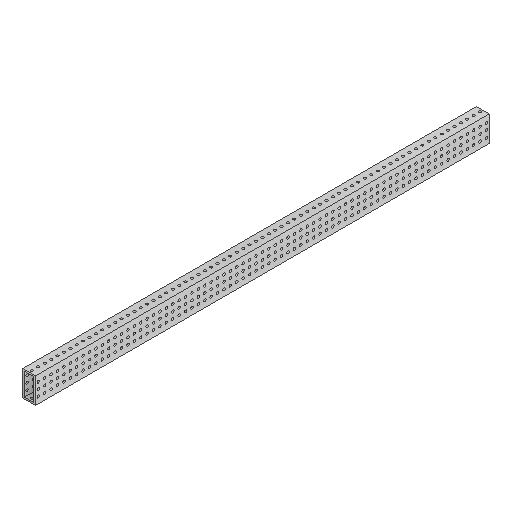
# Autodesk Inventor part: Forja - Base Chassi
Saved by Autodesk Inventor 2027.1 (Build 311270010, 270A)
## iProperties
Created: 2026-05-13
Part Number: Forja - Base Chassi
Material: Genérico
Document SubType Name: Modeling
Designer: djair.oliveira
Density: 1 g/cm^3
Appearance: Padrão
Author: djair.oliveira
Autodesk Inventor part; units mm, degrees
ref_plane "YZ Plane" through (0, 0, 0) normal (1, 0, 0) x (0, 1, 0)
ref_plane "XZ Plane" through (0, 0, 0) normal (0, 1, 0) x (-1, 0, 0)
ref_plane "XY Plane" through (0, 0, 0) normal (0, 0, 1) x (1, 0, 0)
sketch "Esboço1" plane through (0, 0, 0) normal (0, 0, 1) x (1, 0, 0)
  line L0 (12.7, -25.4) -> (-12.7, -25.4)
  line L1 (-12.7, -25.4) -> (-12.7, 25.4)
  line L2 (-12.7, 25.4) -> (12.7, 25.4)
  line L3 (12.7, 25.4) -> (12.7, -25.4)
  line L4 (12.7, -25.4) -> (-12.7, 25.4) construction
  line L5 (-12.7, -25.4) -> (12.7, 25.4) construction
  line L6 (9.525, -22.225) -> (-9.525, -22.225)
  line L7 (-9.525, -22.225) -> (-9.525, 22.225)
  line L8 (-9.525, 22.225) -> (9.525, 22.225)
  line L9 (9.525, 22.225) -> (9.525, -22.225)
  line L10 (9.525, -22.225) -> (-9.525, 22.225) construction
  line L11 (-9.525, -22.225) -> (9.525, 22.225) construction
  point P0 (0, 0)
  dimension "d1" = 3.175
  dimension "d2" = 3.175
  dimension "d3" = 25.4
  dimension "d4" = 50.8
  constraints: 24 end point, 4 midpoint, 4 parallel, 2 horizontal, 2 perpendicular
  measures "d1" distance between parallel lines of L1 L7
  measures "d2" distance between parallel lines of L2 L8
  measures "d3" distance of L1.end L2.end
  measures "d4" distance of L2.end L0.start
extrude "Extrusão1" add sketch "Esboço1" along normal blind 900
sketch "Esboço2" plane through (-12.7, 25.4, 0) normal (0, 1, 0) x (1, 0, 0)
  circle A0 centre (12.7, -450) radius 2.5
  line L0 (0, 0) -> (0, -900) projected
  line L1 (25.4, -900) -> (0, -900) projected
  line L2 (25.4, 0) -> (0, 0) projected
  circle A1 centre (12.7, -462.7) radius 2.5
  circle A2 centre (12.7, -437.3) radius 2.5
  circle A3 centre (12.7, -475.4) radius 2.5
  circle A4 centre (12.7, -424.6) radius 2.5
  circle A5 centre (12.7, -488.1) radius 2.5
  circle A6 centre (12.7, -411.9) radius 2.5
  circle A7 centre (12.7, -500.8) radius 2.5
  circle A8 centre (12.7, -399.2) radius 2.5
  circle A9 centre (12.7, -513.5) radius 2.5
  circle A10 centre (12.7, -386.5) radius 2.5
  circle A11 centre (12.7, -526.2) radius 2.5
  circle A12 centre (12.7, -373.8) radius 2.5
  circle A13 centre (12.7, -538.9) radius 2.5
  circle A14 centre (12.7, -361.1) radius 2.5
  circle A15 centre (12.7, -551.6) radius 2.5
  circle A16 centre (12.7, -348.4) radius 2.5
  circle A17 centre (12.7, -564.3) radius 2.5
  circle A18 centre (12.7, -335.7) radius 2.5
  circle A19 centre (12.7, -577) radius 2.5
  circle A20 centre (12.7, -323) radius 2.5
  circle A21 centre (12.7, -589.7) radius 2.5
  circle A22 centre (12.7, -310.3) radius 2.5
  circle A23 centre (12.7, -602.4) radius 2.5
  circle A24 centre (12.7, -297.6) radius 2.5
  circle A25 centre (12.7, -615.1) radius 2.5
  circle A26 centre (12.7, -284.9) radius 2.5
  circle A27 centre (12.7, -627.8) radius 2.5
  circle A28 centre (12.7, -272.2) radius 2.5
  circle A29 centre (12.7, -640.5) radius 2.5
  circle A30 centre (12.7, -259.5) radius 2.5
  circle A31 centre (12.7, -653.2) radius 2.5
  circle A32 centre (12.7, -246.8) radius 2.5
  circle A33 centre (12.7, -665.9) radius 2.5
  circle A34 centre (12.7, -234.1) radius 2.5
  circle A35 centre (12.7, -678.6) radius 2.5
  circle A36 centre (12.7, -221.4) radius 2.5
  circle A37 centre (12.7, -691.3) radius 2.5
  circle A38 centre (12.7, -208.7) radius 2.5
  circle A39 centre (12.7, -704) radius 2.5
  circle A40 centre (12.7, -196) radius 2.5
  circle A41 centre (12.7, -716.7) radius 2.5
  circle A42 centre (12.7, -183.3) radius 2.5
  circle A43 centre (12.7, -729.4) radius 2.5
  circle A44 centre (12.7, -170.6) radius 2.5
  circle A45 centre (12.7, -742.1) radius 2.5
  circle A46 centre (12.7, -157.9) radius 2.5
  circle A47 centre (12.7, -754.8) radius 2.5
  circle A48 centre (12.7, -145.2) radius 2.5
  circle A49 centre (12.7, -767.5) radius 2.5
  circle A50 centre (12.7, -132.5) radius 2.5
  circle A51 centre (12.7, -780.2) radius 2.5
  circle A52 centre (12.7, -119.8) radius 2.5
  circle A53 centre (12.7, -792.9) radius 2.5
  circle A54 centre (12.7, -107.1) radius 2.5
  circle A55 centre (12.7, -805.6) radius 2.5
  circle A56 centre (12.7, -94.4) radius 2.5
  circle A57 centre (12.7, -818.3) radius 2.5
  circle A58 centre (12.7, -81.7) radius 2.5
  circle A59 centre (12.7, -831) radius 2.5
  circle A60 centre (12.7, -69) radius 2.5
  circle A61 centre (12.7, -843.7) radius 2.5
  circle A62 centre (12.7, -56.3) radius 2.5
  circle A63 centre (12.7, -856.4) radius 2.5
  circle A64 centre (12.7, -43.6) radius 2.5
  circle A65 centre (12.7, -869.1) radius 2.5
  circle A66 centre (12.7, -30.9) radius 2.5
  circle A67 centre (12.7, -881.8) radius 2.5
  circle A68 centre (12.7, -18.2) radius 2.5
  circle A69 centre (12.7, -894.5) radius 2.5
  circle A70 centre (12.7, -5.5) radius 2.5
  point P0 (12.7, 0)
  point P1 (12.7, -900)
  point P2 (12.7, 0)
  point P3 (12.7, 0)
  dimension "d7" = 5
  dimension "d8" = 12.7
  dimension "d9" = 900
  dimension "d10" = 450
  dimension "d13" = 12.7
  constraints: 71 centre point, 3 midpoint, 1 vertical, 140 other
  measures "d7" diameter of A0
  measures "d8" distance from line of L0 A0.centre
  measures "d9" distance of point (12.7, -900) point (12.7, 0)
  measures "d10" distance of point (12.7, 0) A0.centre
  measures "d13" distance of A0.centre A1.centre
extrude "Extrusão2" cut sketch "Esboço2" against normal up to surface (50.8 mm away)
sketch "Esboço3" plane through (12.7, -25.4, 0) normal (1, 0, 0) x (0, 0, -1)
  circle A0 centre (-450, 38.1) radius 2.5
  circle A1 centre (-450, 25.4) radius 2.5
  circle A2 centre (-450, 12.7) radius 2.5
  line L0 (0, 50.8) -> (-900, 50.8) projected
  line L1 (-450, 50.8) -> (-450, 0)
  line L2 (0, 0) -> (-900, 0) projected
  circle A3 centre (-462.7, 38.1) radius 2.5
  circle A4 centre (-462.7, 25.4) radius 2.5
  circle A5 centre (-462.7, 12.7) radius 2.5
  circle A6 centre (-437.3, 38.1) radius 2.5
  circle A7 centre (-437.3, 25.4) radius 2.5
  circle A8 centre (-437.3, 12.7) radius 2.5
  circle A9 centre (-475.4, 38.1) radius 2.5
  circle A10 centre (-475.4, 25.4) radius 2.5
  circle A11 centre (-475.4, 12.7) radius 2.5
  circle A12 centre (-424.6, 38.1) radius 2.5
  circle A13 centre (-424.6, 25.4) radius 2.5
  circle A14 centre (-424.6, 12.7) radius 2.5
  circle A15 centre (-488.1, 38.1) radius 2.5
  circle A16 centre (-488.1, 25.4) radius 2.5
  circle A17 centre (-488.1, 12.7) radius 2.5
  circle A18 centre (-411.9, 38.1) radius 2.5
  circle A19 centre (-411.9, 25.4) radius 2.5
  circle A20 centre (-411.9, 12.7) radius 2.5
  circle A21 centre (-500.8, 38.1) radius 2.5
  circle A22 centre (-500.8, 25.4) radius 2.5
  circle A23 centre (-500.8, 12.7) radius 2.5
  circle A24 centre (-399.2, 38.1) radius 2.5
  circle A25 centre (-399.2, 25.4) radius 2.5
  circle A26 centre (-399.2, 12.7) radius 2.5
  circle A27 centre (-513.5, 38.1) radius 2.5
  circle A28 centre (-513.5, 25.4) radius 2.5
  circle A29 centre (-513.5, 12.7) radius 2.5
  circle A30 centre (-386.5, 38.1) radius 2.5
  circle A31 centre (-386.5, 25.4) radius 2.5
  circle A32 centre (-386.5, 12.7) radius 2.5
  circle A33 centre (-526.2, 38.1) radius 2.5
  circle A34 centre (-526.2, 25.4) radius 2.5
  circle A35 centre (-526.2, 12.7) radius 2.5
  circle A36 centre (-373.8, 38.1) radius 2.5
  circle A37 centre (-373.8, 25.4) radius 2.5
  circle A38 centre (-373.8, 12.7) radius 2.5
  circle A39 centre (-538.9, 38.1) radius 2.5
  circle A40 centre (-538.9, 25.4) radius 2.5
  circle A41 centre (-538.9, 12.7) radius 2.5
  circle A42 centre (-361.1, 38.1) radius 2.5
  circle A43 centre (-361.1, 25.4) radius 2.5
  circle A44 centre (-361.1, 12.7) radius 2.5
  circle A45 centre (-551.6, 38.1) radius 2.5
  circle A46 centre (-551.6, 25.4) radius 2.5
  circle A47 centre (-551.6, 12.7) radius 2.5
  circle A48 centre (-348.4, 38.1) radius 2.5
  circle A49 centre (-348.4, 25.4) radius 2.5
  circle A50 centre (-348.4, 12.7) radius 2.5
  circle A51 centre (-564.3, 38.1) radius 2.5
  circle A52 centre (-564.3, 25.4) radius 2.5
  circle A53 centre (-564.3, 12.7) radius 2.5
  circle A54 centre (-335.7, 38.1) radius 2.5
  circle A55 centre (-335.7, 25.4) radius 2.5
  circle A56 centre (-335.7, 12.7) radius 2.5
  circle A57 centre (-577, 38.1) radius 2.5
  circle A58 centre (-577, 25.4) radius 2.5
  circle A59 centre (-577, 12.7) radius 2.5
  circle A60 centre (-323, 38.1) radius 2.5
  circle A61 centre (-323, 25.4) radius 2.5
  circle A62 centre (-323, 12.7) radius 2.5
  circle A63 centre (-589.7, 38.1) radius 2.5
  circle A64 centre (-589.7, 25.4) radius 2.5
  circle A65 centre (-589.7, 12.7) radius 2.5
  circle A66 centre (-310.3, 38.1) radius 2.5
  circle A67 centre (-310.3, 25.4) radius 2.5
  circle A68 centre (-310.3, 12.7) radius 2.5
  circle A69 centre (-602.4, 38.1) radius 2.5
  circle A70 centre (-602.4, 25.4) radius 2.5
  circle A71 centre (-602.4, 12.7) radius 2.5
  circle A72 centre (-297.6, 38.1) radius 2.5
  circle A73 centre (-297.6, 25.4) radius 2.5
  circle A74 centre (-297.6, 12.7) radius 2.5
  circle A75 centre (-615.1, 38.1) radius 2.5
  circle A76 centre (-615.1, 25.4) radius 2.5
  circle A77 centre (-615.1, 12.7) radius 2.5
  circle A78 centre (-284.9, 38.1) radius 2.5
  circle A79 centre (-284.9, 25.4) radius 2.5
  circle A80 centre (-284.9, 12.7) radius 2.5
  circle A81 centre (-627.8, 38.1) radius 2.5
  circle A82 centre (-627.8, 25.4) radius 2.5
  circle A83 centre (-627.8, 12.7) radius 2.5
  circle A84 centre (-272.2, 38.1) radius 2.5
  circle A85 centre (-272.2, 25.4) radius 2.5
  circle A86 centre (-272.2, 12.7) radius 2.5
  circle A87 centre (-640.5, 38.1) radius 2.5
  circle A88 centre (-640.5, 25.4) radius 2.5
  circle A89 centre (-640.5, 12.7) radius 2.5
  circle A90 centre (-259.5, 38.1) radius 2.5
  circle A91 centre (-259.5, 25.4) radius 2.5
  circle A92 centre (-259.5, 12.7) radius 2.5
  circle A93 centre (-653.2, 38.1) radius 2.5
  circle A94 centre (-653.2, 25.4) radius 2.5
  circle A95 centre (-653.2, 12.7) radius 2.5
  circle A96 centre (-246.8, 38.1) radius 2.5
  circle A97 centre (-246.8, 25.4) radius 2.5
  circle A98 centre (-246.8, 12.7) radius 2.5
  circle A99 centre (-665.9, 38.1) radius 2.5
  circle A100 centre (-665.9, 25.4) radius 2.5
  circle A101 centre (-665.9, 12.7) radius 2.5
  circle A102 centre (-234.1, 38.1) radius 2.5
  circle A103 centre (-234.1, 25.4) radius 2.5
  circle A104 centre (-234.1, 12.7) radius 2.5
  circle A105 centre (-678.6, 38.1) radius 2.5
  circle A106 centre (-678.6, 25.4) radius 2.5
  circle A107 centre (-678.6, 12.7) radius 2.5
  circle A108 centre (-221.4, 38.1) radius 2.5
  circle A109 centre (-221.4, 25.4) radius 2.5
  circle A110 centre (-221.4, 12.7) radius 2.5
  circle A111 centre (-691.3, 38.1) radius 2.5
  circle A112 centre (-691.3, 25.4) radius 2.5
  circle A113 centre (-691.3, 12.7) radius 2.5
  circle A114 centre (-208.7, 38.1) radius 2.5
  circle A115 centre (-208.7, 25.4) radius 2.5
  circle A116 centre (-208.7, 12.7) radius 2.5
  circle A117 centre (-704, 38.1) radius 2.5
  circle A118 centre (-704, 25.4) radius 2.5
  circle A119 centre (-704, 12.7) radius 2.5
  circle A120 centre (-196, 38.1) radius 2.5
  circle A121 centre (-196, 25.4) radius 2.5
  circle A122 centre (-196, 12.7) radius 2.5
  circle A123 centre (-716.7, 38.1) radius 2.5
  circle A124 centre (-716.7, 25.4) radius 2.5
  circle A125 centre (-716.7, 12.7) radius 2.5
  circle A126 centre (-183.3, 38.1) radius 2.5
  circle A127 centre (-183.3, 25.4) radius 2.5
  circle A128 centre (-183.3, 12.7) radius 2.5
  circle A129 centre (-729.4, 38.1) radius 2.5
  circle A130 centre (-729.4, 25.4) radius 2.5
  circle A131 centre (-729.4, 12.7) radius 2.5
  circle A132 centre (-170.6, 38.1) radius 2.5
  circle A133 centre (-170.6, 25.4) radius 2.5
  circle A134 centre (-170.6, 12.7) radius 2.5
  circle A135 centre (-742.1, 38.1) radius 2.5
  circle A136 centre (-742.1, 25.4) radius 2.5
  circle A137 centre (-742.1, 12.7) radius 2.5
  circle A138 centre (-157.9, 38.1) radius 2.5
  circle A139 centre (-157.9, 25.4) radius 2.5
  circle A140 centre (-157.9, 12.7) radius 2.5
  circle A141 centre (-754.8, 38.1) radius 2.5
  circle A142 centre (-754.8, 25.4) radius 2.5
  circle A143 centre (-754.8, 12.7) radius 2.5
  circle A144 centre (-145.2, 38.1) radius 2.5
  circle A145 centre (-145.2, 25.4) radius 2.5
  circle A146 centre (-145.2, 12.7) radius 2.5
  circle A147 centre (-767.5, 38.1) radius 2.5
  circle A148 centre (-767.5, 25.4) radius 2.5
  circle A149 centre (-767.5, 12.7) radius 2.5
  circle A150 centre (-132.5, 38.1) radius 2.5
  circle A151 centre (-132.5, 25.4) radius 2.5
  circle A152 centre (-132.5, 12.7) radius 2.5
  circle A153 centre (-780.2, 38.1) radius 2.5
  circle A154 centre (-780.2, 25.4) radius 2.5
  circle A155 centre (-780.2, 12.7) radius 2.5
  circle A156 centre (-119.8, 38.1) radius 2.5
  circle A157 centre (-119.8, 25.4) radius 2.5
  circle A158 centre (-119.8, 12.7) radius 2.5
  circle A159 centre (-792.9, 38.1) radius 2.5
  circle A160 centre (-792.9, 25.4) radius 2.5
  circle A161 centre (-792.9, 12.7) radius 2.5
  circle A162 centre (-107.1, 38.1) radius 2.5
  circle A163 centre (-107.1, 25.4) radius 2.5
  circle A164 centre (-107.1, 12.7) radius 2.5
  circle A165 centre (-805.6, 38.1) radius 2.5
  circle A166 centre (-805.6, 25.4) radius 2.5
  circle A167 centre (-805.6, 12.7) radius 2.5
  circle A168 centre (-94.4, 38.1) radius 2.5
  circle A169 centre (-94.4, 25.4) radius 2.5
  circle A170 centre (-94.4, 12.7) radius 2.5
  circle A171 centre (-818.3, 38.1) radius 2.5
  circle A172 centre (-818.3, 25.4) radius 2.5
  circle A173 centre (-818.3, 12.7) radius 2.5
  circle A174 centre (-81.7, 38.1) radius 2.5
  circle A175 centre (-81.7, 25.4) radius 2.5
  circle A176 centre (-81.7, 12.7) radius 2.5
  circle A177 centre (-831, 38.1) radius 2.5
  circle A178 centre (-831, 25.4) radius 2.5
  circle A179 centre (-831, 12.7) radius 2.5
  circle A180 centre (-69, 38.1) radius 2.5
  circle A181 centre (-69, 25.4) radius 2.5
  circle A182 centre (-69, 12.7) radius 2.5
  circle A183 centre (-843.7, 38.1) radius 2.5
  circle A184 centre (-843.7, 25.4) radius 2.5
  circle A185 centre (-843.7, 12.7) radius 2.5
  circle A186 centre (-56.3, 38.1) radius 2.5
  circle A187 centre (-56.3, 25.4) radius 2.5
  circle A188 centre (-56.3, 12.7) radius 2.5
  circle A189 centre (-856.4, 38.1) radius 2.5
  circle A190 centre (-856.4, 25.4) radius 2.5
  circle A191 centre (-856.4, 12.7) radius 2.5
  circle A192 centre (-43.6, 38.1) radius 2.5
  circle A193 centre (-43.6, 25.4) radius 2.5
  circle A194 centre (-43.6, 12.7) radius 2.5
  circle A195 centre (-869.1, 38.1) radius 2.5
  circle A196 centre (-869.1, 25.4) radius 2.5
  circle A197 centre (-869.1, 12.7) radius 2.5
  circle A198 centre (-30.9, 38.1) radius 2.5
  circle A199 centre (-30.9, 25.4) radius 2.5
  circle A200 centre (-30.9, 12.7) radius 2.5
  circle A201 centre (-881.8, 38.1) radius 2.5
  circle A202 centre (-881.8, 25.4) radius 2.5
  circle A203 centre (-881.8, 12.7) radius 2.5
  circle A204 centre (-18.2, 38.1) radius 2.5
  circle A205 centre (-18.2, 25.4) radius 2.5
  circle A206 centre (-18.2, 12.7) radius 2.5
  circle A207 centre (-894.5, 38.1) radius 2.5
  circle A208 centre (-894.5, 25.4) radius 2.5
  circle A209 centre (-894.5, 12.7) radius 2.5
  circle A210 centre (-5.5, 38.1) radius 2.5
  circle A211 centre (-5.5, 25.4) radius 2.5
  circle A212 centre (-5.5, 12.7) radius 2.5
  point P0 (0, 25.4)
  dimension "d20" = 5
  dimension "d21" = 25.4
  dimension "d22" = 12.7
  dimension "d23" = 12.7
  dimension "d26" = 12.7
  constraints: 213 centre point, 2 end point, 2 equal radius, 2 midpoint, 2 vertical alignment, 1 horizontal, 1 point on line, 420 other
  measures "d20" diameter of A1
  measures "d21" distance from line of L0 A1.centre
  measures "d22" distance of A0.centre A1.centre
  measures "d23" distance of A2.centre A1.centre
  measures "d26" distance of A0.centre A3.centre
extrude "Extrusão3" cut sketch "Esboço3" against normal up to surface (25.4 mm away)
equation "\"d2\" = d1"
equation "\"d10\" = 0.5 * d9"
equation "\"d23\" = d22"
